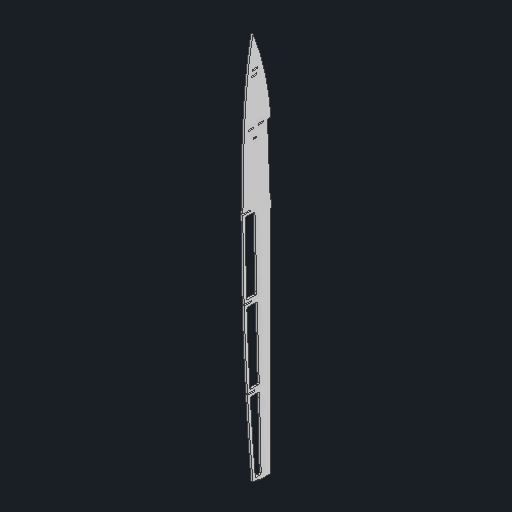
# Autodesk Inventor part: stringer
Saved by Autodesk Inventor 2023 (Build 270158030, 158C)
## iProperties
Created: 2022-03-21
Part Number: stringer
Material: Generic
Document SubType Name: Modeling
Designer: kardo
Density: 1 g/cm^3
Appearance: Default
Mass: 50.8397 g
Surface Area: 402.853 cm^2
Volume: 50.8397 cm^3
Author: kardo
Autodesk Inventor part; units mm, degrees
ref_plane "YZ Plane" through (0, 0, 0) normal (1, 0, 0) x (0, 1, 0)
ref_plane "XZ Plane" through (0, 0, 0) normal (0, 1, 0) x (-1, 0, 0)
ref_plane "XY Plane" through (0, 0, 0) normal (0, 0, 1) x (1, 0, 0)
derived "parameters_frame.ipt"
derived "surface_body.ipt"
sketch "sk_long_outer" plane through (0, 0, 0) normal (1, 0, 0) x (0, 1, 0)
  line L0 (-363, 107.6209) -> (-363, -224.5198) construction
  line L1 (237, 107.6209) -> (237, -224.5198) construction
  line L2 (-483, 54.4) -> (357, 54.4) construction
  line L3 (-483, 0) -> (357, 0) construction
  line L4 (0, 107.6209) -> (0, -224.5198) construction
  line L5 (0, 8.704) -> (-363, 9.792)
  line L6 (-363, 9.792) -> (-363, 39.712)
  line L7 (-363, 39.712) -> (0, 54.4)
  line L8 (0, 54.4) -> (237, 36.448)
  line L9 (0, 0) -> (111.39, 7.7891)
  line L10 (111.39, 7.7891) -> (237, 36.448)
  line L11 (0, 8.704) -> (0, 0)
  line L12 (0, 8.704) -> (111.0257, 12.9988)
  line L13 (111.0257, 12.9988) -> (111.39, 7.7891)
sketch "sk_rail_sponson_tunnel" plane through (81.12, 0, 0) normal (1, 0, 0) x (0, 1, 0)
  line L0 (0, 0) -> (111.39, 7.7891)
  line L1 (101.5485, 148.5297) -> (128.7646, -240.679) construction
  spline S0 degree 2 poles (111.39, 7.7891) (176.0348, 12.3096) (237, 36.448) knots 0 0 0 1 1 1
sketch "sk_rail_top_tunnel" plane through (81.12, 0, 0) normal (1, 0, 0) x (0, 1, 0)
  line L0 (237, 107.6209) -> (237, -224.5198) construction
  line L1 (0, 107.6209) -> (0, -224.5198) construction
  line L2 (-363, 107.6209) -> (-363, -224.5198) construction
  line L3 (-363, 0) -> (0, 0) construction
  line L4 (-181.5, 48.8998) -> (-181.5, 0) construction
  line L5 (0, 52.89) -> (31.284, 52.89) construction
  line L6 (31.284, 52.89) -> (68.256, 47.0555) construction
  line L7 (68.256, 47.0555) -> (94.8, 37.536) construction
  line L8 (94.8, 107.6209) -> (94.8, -224.5198) construction
  line L9 (0, 52.89) -> (237, 52.89) construction
  line L10 (-488.1035, 0) -> (361.1125, 0) construction
  spline S0 degree 3 poles (0, 52.89) (86.3106, 52.89) (181.3207, 49.5034) (237, 36.448) knots 0 0 0 0 1 1 1 1
  spline S1 degree 3 poles (0, 52.89) (31.284, 52.89) (68.256, 47.0555) (94.8, 37.536) knots 1 1 1 1 2 2 2 2
  spline S2 degree 4 poles (-363, 37.4293) (-272.3626, 45.1427) (-181.5879, 49.7528) (-90.8131, 52.89) (0, 52.89) knots 0 0 0 0 0 1 1 1 1 1
  point P0 (142.2, 48.7795)
  point P1 (94.8, 28.832)
  point P2 (-242.0001, 45.8501)
  point P3 (-120.9999, 51.0063)
sketch "sk_rail_bottom_tunnel" plane through (81.12, 0, 0) normal (1, 0, 0) x (0, 1, 0)
  line L0 (-254.1001, 21.0191) -> (9.48, 28.5282)
  arc A0 (30.81, 28.832) -> (9.48, 28.5282) centre (30.81, -720.1791) ccw
  line L1 (30.81, 28.832) -> (94.8, 28.832)
  arc A1 (-275.8801, 20.463) -> (-254.1001, 21.0191) centre (-359.1231, 3707.4463) ccw
  line L2 (-363, 18.496) -> (-275.8801, 20.463)
  point P0 (0, 0)
ref_plane "plane_middle" through (0, 0, 0) normal (0, 1, 0) x (-1, 0, 0)
ref_plane "plane_tunnel_right" through (81.12, 0, 0) normal (1, 0, 0) x (0, 1, 0)
ref_plane "plane_tail_1" through (0, -120.9999, 0) normal (0, 1, 0) x (-1, 0, 0)
ref_plane "plane_tail_2" through (0, -242.0001, 0) normal (0, 1, 0) x (-1, 0, 0)
derived "stencil_frame.ipt"
sketch "sk_joint_locations" plane through (81.12, 0, 0) normal (1, 0, 0) x (0, 1, 0)
  line L0 (0, 0) -> (111.39, 7.7891) construction
  line L1 (30.81, 28.832) -> (94.8, 28.832) construction
  arc A0 (30.81, 28.832) -> (9.48, 28.5282) centre (30.81, -720.1791) ccw construction
  line L2 (-254.1001, 21.0191) -> (9.48, 28.5282) construction
  line L3 (-363, 18.496) -> (-275.8801, 20.463) construction
  arc A1 (-275.8801, 20.463) -> (-254.1001, 21.0191) centre (-359.1231, 3707.4463) ccw construction
  line L4 (-215.9778, 4689.3669) -> (255.6105, -2054.6605) construction
  line L5 (-242.0001, 4666.1952) -> (-242.0001, -2045.0469) construction
  line L6 (-120.9999, 4666.1952) -> (-120.9999, -2045.0469) construction
  line L7 (-363, 4666.1952) -> (-363, -2045.0469) construction
  line L8 (0, 4666.1952) -> (0, -2045.0469) construction
  line L9 (554.3783, 47.5311) -> (-618.9921, 6.5561) construction
  line L10 (-688.3759, -28.2606) -> (714.4996, 69.838) construction
  line L11 (178.2183, 30.3929) -> (177.9391, 38.388) construction
  line L12 (185.9231, 36.8959) -> (186.4825, 28.8959) construction
  line L13 (0, 8.704) -> (111.0257, 12.9988) construction
  line L14 (-242.0001, 45.8501) -> (-242.0001, 21.3638) construction
  line L15 (-363, 37.4293) -> (-363, 18.496) construction
  line L16 (-120.9999, 51.0063) -> (-120.9999, 24.811) construction
  line L17 (0, 52.89) -> (0, 28.2581) construction
  line L18 (108.3896, 50.6971) -> (108.9168, 43.1574) construction
  line L19 (109.444, 35.6178) -> (108.9168, 43.1574) construction
  line L20 (109.444, 35.6178) -> (109.9713, 28.0781) construction
  line L21 (109.9713, 28.0781) -> (110.4985, 20.5385) construction
  line L22 (110.4985, 20.5385) -> (111.0257, 12.9988) construction
  line L23 (0, 8.704) -> (0, 0) construction
  spline S0 degree 4 poles (-363, 37.4293) (-272.3626, 45.1427) (-181.5879, 49.7528) (-90.8131, 52.89) (0, 52.89) knots 0 0 0 0 0 1 1 1 1 1
  spline S1 degree 3 poles (0, 52.89) (86.3106, 52.89) (181.3207, 49.5034) (237, 36.448) knots 0 0 0 0 1 1 1 1
  spline S2 degree 2 poles (111.39, 7.7891) (176.0348, 12.3096) (237, 36.448) knots 0 0 0 1 1 1
  line L24 (94.8, 37.536) -> (94.8, 28.832) construction
  line L25 (94.8, 35.548) -> (94.8, 30.82) construction
  point P0 (178.0787, 34.3904)
  point P1 (186.2028, 32.8959)
  point P2 (-363, 27.9627)
  point P3 (-242.0001, 33.6069)
  point P4 (-120.9999, 37.9086)
  point P5 (0, 40.5741)
  point P6 (94.8, 33.184)
sketch "sk_stringer_base" plane through (81.12, 0, 0) normal (1, 0, 0) x (0, 1, 0)
  line L0 (0, 8.704) -> (-363, 9.792) construction
  spline S0 degree 4 poles (-363, 37.4293) (-272.3626, 45.1427) (-181.5879, 49.7528) (-90.8131, 52.89) (0, 52.89) knots 0 0 0 0 0 1 1 1 1 1 construction
  spline S1 degree 3 poles (0, 52.89) (31.284, 52.89) (68.256, 47.0555) (94.8, 37.536) knots 1 1 1 1 2 2 2 2 construction
  spline S2 degree 3 poles (0, 52.89) (86.3106, 52.89) (181.3207, 49.5034) (237, 36.448) knots 0 0 0 0 1 1 1 1 construction
  spline S3 degree 2 poles (111.39, 7.7891) (176.0348, 12.3096) (237, 36.448) knots 0 0 0 1 1 1 construction
  line L1 (0, 0) -> (111.39, 7.7891) construction
  line L2 (-363, 18.496) -> (-275.8801, 20.463) construction
  arc A0 (-275.8801, 20.463) -> (-254.1001, 21.0191) centre (-359.1231, 3707.4463) ccw construction
  line L3 (-254.1001, 21.0191) -> (9.48, 28.5282) construction
  arc A1 (30.81, 28.832) -> (9.48, 28.5282) centre (30.81, -720.1791) ccw construction
  line L4 (30.81, 28.832) -> (94.8, 28.832) construction
  line L5 (0, 4592.9714) -> (0, -1605.7041) construction
  line L6 (-363, 27.9627) -> (-363, 9.792)
  line L7 (-363, 9.792) -> (0, 8.704)
  line L8 (109.3112, 8.8467) -> (108.9425, 14.1191)
  line L9 (0, 8.704) -> (0, 9.904)
  line L10 (0, 9.904) -> (108.9425, 14.1191)
  line L11 (-363, 27.9627) -> (-361, 27.9627)
  line L12 (-361, 27.9627) -> (-361, 36.3947)
  line L13 (-242.0001, 33.6069) -> (-240.0001, 33.6069)
  line L14 (-240.0001, 33.6069) -> (-240.0001, 44.7587)
  line L15 (-242.0001, 33.6069) -> (-242.0001, 44.6482)
  line L16 (-120.9999, 37.9086) -> (-120.9999, 49.8057)
  line L17 (-120.9999, 37.9086) -> (-118.9999, 37.9086)
  line L18 (-118.9999, 37.9086) -> (-118.9999, 49.8649)
  line L19 (0, 51.69) -> (0, 40.5741)
  line L20 (0, 40.5741) -> (2, 40.5741)
  line L21 (2, 40.5741) -> (2, 51.6894)
  line L22 (108.9168, 43.1574) -> (109.444, 35.6178)
  line L23 (109.444, 35.6178) -> (107.4489, 35.4783)
  line L24 (107.4489, 35.4783) -> (106.9217, 43.0179)
  line L25 (106.9217, 43.0179) -> (108.9168, 43.1574)
  line L26 (109.9713, 28.0781) -> (107.9761, 27.9386)
  line L27 (107.9761, 27.9386) -> (108.5034, 20.399)
  line L28 (108.5034, 20.399) -> (110.4985, 20.5385)
  line L29 (109.9713, 28.0781) -> (110.4985, 20.5385)
  line L30 (177.9391, 38.388) -> (178.2183, 30.3929)
  line L31 (185.9231, 36.8959) -> (186.4825, 28.8959)
  line L32 (186.4825, 28.8959) -> (184.4874, 28.7564)
  line L33 (184.4874, 28.7564) -> (183.9279, 36.7564)
  line L34 (183.9279, 36.7564) -> (185.9231, 36.8959)
  line L35 (177.9391, 38.388) -> (175.9404, 38.3182)
  line L36 (175.9404, 38.3182) -> (176.2196, 30.3231)
  line L37 (176.2196, 30.3231) -> (178.2183, 30.3929)
  line L38 (111.3063, 8.9862) -> (109.3112, 8.8467)
  line L39 (92.8, 35.548) -> (94.8, 35.548)
  line L40 (94.8, 35.548) -> (94.8, 30.82)
  line L41 (94.8, 30.82) -> (92.8, 30.82)
  line L42 (92.8, 30.82) -> (92.8, 35.548)
  spline S4 degree 5 poles (-361, 36.3947) (-288.9726, 42.4857) (-216.7915, 46.7542) (-144.5684, 49.8252) (-72.2845, 51.6901) (0, 51.69) knots 0 0 0 0 0 0 1 1 1 1 1 1
  spline S5 degree 5 poles (0, 51.69) (13.1181, 51.69) (26.2363, 51.6248) (39.354, 51.4874) (65.3463, 51.0551) (91.3298, 50.254) (104.1978, 49.754) (128.8047, 48.5691) (153.3792, 46.8416) (165.0971, 45.8705) (186.544, 43.7678) (207.8948, 40.8506) (217.5643, 39.3125) (227.1954, 37.5137) (236.7261, 35.2797) knots 0 0 0 0 0 0 0.275935 0.275935 0.275935 0.546799 0.546799 0.546799 0.794097 0.794097 0.794097 1 1 1 1 1 1
  spline S6 degree 5 poles (236.5582, 37.5637) (212.5733, 28.0675) (187.8895, 20.337) (162.6364, 14.5485) (137.0398, 10.7859) (111.3063, 8.9862) knots 0 0 0 0 0 0 1 1 1 1 1 1
  point P0 (232.9228, 36.1431)
  point P1 (111.0257, 12.9988)
  dimension "d4" = 1.2
  dimension "d14" = 1.2
  dimension "d8" = 1.2
  dimension "d9" = 2
  dimension "d11" = 2
  dimension "d16" = 2
  dimension "d17" = 1.2
  constraints: 74 end point, 12 perpendicular, 7 vertical, 6 equal length, 6 parallel, 2 coincident, 2 collinear, 2 horizontal, 18 other
  measures "d8" distance of L7.end L9.end
  measures "d9" distance of L6.start L11.end
  measures "d11" distance of L19.end L20.end
  measures "d16" distance between parallel lines of L40 L42
  measures "d17" distance from line of point (111.026, 12.999) L10
extrude "thicken" add sketch "sk_stringer_base" along normal blind 3 contours L11 L12 S4 L15 L13 L14 L16 L17 L18 L19 L20 L21 S5 S6 L38 L8 L10 L9 L7 L6
sketch "sk_cut_weight" plane through (81.12, 0, 0) normal (1, 0, 0) x (0, 1, 0)
  spline S0 degree 4 poles (-363, 37.4293) (-272.3626, 45.1427) (-181.5879, 49.7528) (-90.8131, 52.89) (0, 52.89) knots 0 0 0 0 0 1 1 1 1 1 construction
  spline S1 degree 3 poles (0, 52.89) (31.284, 52.89) (68.256, 47.0555) (94.8, 37.536) knots 1 1 1 1 2 2 2 2 construction
  line L0 (30.81, 28.832) -> (94.8, 28.832) construction
  arc A0 (30.81, 28.832) -> (9.48, 28.5282) centre (30.81, -720.1791) ccw construction
  line L1 (-254.1001, 21.0191) -> (9.48, 28.5282) construction
  arc A1 (-275.8801, 20.463) -> (-254.1001, 21.0191) centre (-359.1231, 3707.4463) ccw construction
  line L2 (-363, 18.496) -> (-275.8801, 20.463) construction
  line L3 (94.8, 37.536) -> (94.8, 28.832) construction
  line L4 (89.01, 34.032) -> (30.81, 34.032)
  arc A2 (30.81, 34.032) -> (9.3319, 33.7261) centre (30.81, -720.1791) ccw
  line L5 (9.3319, 33.7261) -> (-254.2482, 26.217)
  arc A3 (-275.9975, 25.6616) -> (-254.2482, 26.217) centre (-359.1231, 3707.4463) ccw
  line L6 (-275.9975, 25.6616) -> (-357, 23.8328)
  line L7 (-363, 18.496) -> (-363, 37.4293) construction
  line L8 (-361, 46.328) -> (-361, 7.7109) construction
  line L9 (-240.0001, 59.5201) -> (-240.0001, 2.898) construction
  line L10 (-118.9999, 68.9991) -> (-118.9999, 15.2181) construction
  line L11 (0, 4592.9714) -> (0, -1605.7041) construction
  line L12 (-242.0001, 4592.9714) -> (-242.0001, -1605.7041) construction
  line L13 (-120.9999, 4592.9714) -> (-120.9999, -1605.7041) construction
  line L14 (-357, 23.8328) -> (-357, 32.7168)
  line L15 (-246.0001, 40.4184) -> (-246.0001, 26.4519)
  line L16 (-236.0001, 40.9712) -> (-236.0001, 26.7368)
  line L17 (-124.9999, 45.683) -> (-124.9999, 29.8991)
  line L18 (-114.9999, 45.9789) -> (-114.9999, 30.184)
  line L19 (-4, 47.6877) -> (-4, 33.3463)
  spline S2 degree 5 poles (-357, 32.7168) (-285.7663, 38.6671) (-214.3855, 42.8518) (-142.963, 45.8644) (-71.4819, 47.6901) (0, 47.69) knots 0 0 0 0 0 0 1 1 1 1 1 1
  spline S3 degree 5 poles (0, 47.69) (9.7143, 47.6897) (19.4272, 47.2129) (29.1127, 46.3746) (47.0689, 44.1714) (64.8269, 40.7273) (72.9831, 38.8494) (81.0702, 36.6635) (89.0099, 34.0319) knots 0 0 0 0 0 0 0.53732 0.53732 0.53732 1 1 1 1 1 1
  point P0 (0, 0)
  dimension "d20" = 5.2
  dimension "d21" = 2
  dimension "d22" = 2
  dimension "d23" = 2
  dimension "d25" = 4
  dimension "d26" = 4
  dimension "d27" = 4
  dimension "d28" = 4
  dimension "d29" = 4
  dimension "d30" = 4
  constraints: 29 end point, 10 parallel, 5 point on line, 4 point on circle, 2 centre point, 16 other
  measures "d21" distance between parallel lines of L7 L8
  measures "d22" distance between parallel lines of L12 L9
  measures "d23" distance between parallel lines of L13 L10
  measures "d25" distance between parallel lines of L8 L14
  measures "d26" distance between parallel lines of L12 L15
  measures "d27" distance between parallel lines of L9 L16
  measures "d28" distance between parallel lines of L17 L13
  measures "d29" distance between parallel lines of L18 L10
  measures "d30" distance between parallel lines of L19 L11
extrude "cut_weight" cut sketch "sk_cut_weight" along normal through all both and the other way through all contours L19 L5 L18 S2 | L17 L5 L16 S2 | L15 L5 A3 L6 L14 S2
fillet "rounding" radius 2 12 edges at (82.62, -4, 33.3463) (82.62, -4, 47.6877) (82.62, -124.9999, 45.683) (82.62, -246.0001, 40.4184) (82.62, -246.0001, 26.4519) (82.62, -124.9999, 29.8991) (82.62, -357, 23.8328) (82.62, -236.0001, 26.7368) (82.62, -114.9999, 30.184) (82.62, -114.9999, 45.9789) (82.62, -236.0001, 40.9712) (82.62, -357, 32.7168)
equation "\"d4\" = shell_thickness"
equation "\"d14\" = shell_thickness"
equation "\"d8\" = shell_thickness"
equation "\"d9\" = bulkhead_thickness"
equation "\"d11\" = bulkhead_thickness"
equation "\"d16\" = bulkhead_thickness"
equation "\"d17\" = shell_thickness"
equation "\"d12\" = stringer_thickness"
equation "\"d20\" = bulkhead_inset + shell_thickness"
equation "\"d21\" = bulkhead_thickness"
equation "\"d22\" = bulkhead_thickness"
equation "\"d23\" = bulkhead_thickness"
equation "\"d25\" = bulkhead_inset"
equation "\"d26\" = bulkhead_inset"
equation "\"d27\" = bulkhead_inset"
equation "\"d28\" = bulkhead_inset"
equation "\"d29\" = bulkhead_inset"
equation "\"d30\" = bulkhead_inset"
equation "\"d34\" = 0.5 * bulkhead_inset"
equation "\"shell_thickness\" = 1.2"
equation "\"bulkhead_thickness\" = 2"
equation "\"stringer_thickness\" = 3"
equation "\"bulkhead_inset\" = 4"
body "Solid1"
